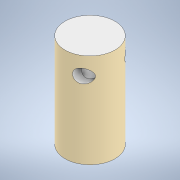
# Autodesk Inventor part: W520inferior
Saved by Autodesk Inventor 2020 (Build 240168000, 168)
## iProperties
Created: 2021-10-16
Part Number: W520inferior
Material: Genérico
Document SubType Name: Modeling
Designer: DANIEL
Density: 1 g/cm^3
Appearance: Suave - Blanco
Author: DANIEL
Autodesk Inventor part; units mm, degrees
ref_plane "YZ Plane" through (0, 0, 0) normal (1, 0, 0) x (0, 1, 0)
ref_plane "XZ Plane" through (0, 0, 0) normal (0, 1, 0) x (-1, 0, 0)
sketch "Boceto1" plane through (0, 0, 0) normal (0, 1, 0) x (-1, 0, 0)
  circle A0 centre (0, 0) radius 10.95
  dimension "d0" = 21.9
  constraints: 1 centre point, 1 coincident
  measures "d0" diameter of A0
extrude "Extrusión1" add sketch "Boceto1" along normal blind 146.5
sketch "Boceto2" plane through (0, 0, 0) normal (0, -1, 0) x (1, 0, 0)
  circle A0 centre (3.4074, 3.75) radius 3
  circle A1 centre (3.4074, -3.75) radius 3
  circle A2 centre (-4.9805, 0) radius 3.5
  point P0 (0, 0)
  dimension "d3" = 6
  dimension "d4" = 6
  dimension "d5" = 7
  dimension "d" = 7.5
  dimension "d7" = 3.75
  constraints: 3 centre point
  measures "d3" diameter of A0
  measures "d4" diameter of A1
  measures "d5" diameter of A2
  measures "d" distance of A0.centre A1.centre
  measures "d7" vertical distance of A1.centre point (0, 0)
extrude "Extrusión2" cut sketch "Boceto2" against normal blind 40.5
sketch "Boceto4" plane through (0, 0, 0) normal (0, -1, 0) x (1, 0, 0)
  circle A0 centre (0, 0) radius 10.95
  circle A1 centre (0, 0) radius 11
  dimension "d10" = 22
  constraints: 2 centre point, 2 coincident
  measures "d10" diameter of A1
extrude "Extrusión3" add sketch "Boceto4" against normal blind 41.5
sketch "Boceto5" plane through (0, 146.5, 0) normal (0, 1, 0) x (1, 0, 0)
  circle A0 centre (0, 0) radius 10.95
  constraints: 1 centre point, 1 coincident
extrude "Extrusión4" cut sketch "Boceto5" against normal blind 105
ref_plane "Plano de trabajo1" through (0, 0, 0) normal (0, 0, 1) x (1, 0, 0)
sketch "Boceto6" plane through (0, 0, 0) normal (0, 0, 1) x (1, 0, 0)
  circle A0 centre (5.8998, 33.6799) radius 3
  point P0 (0, 0)
  dimension "d16" = 6
  constraints: 1 centre point
  measures "d16" diameter of A0
extrude "Extrusión5" cut sketch "Boceto6" along normal mid plane 22
equation "\"d7\" = 0.5 * d"
